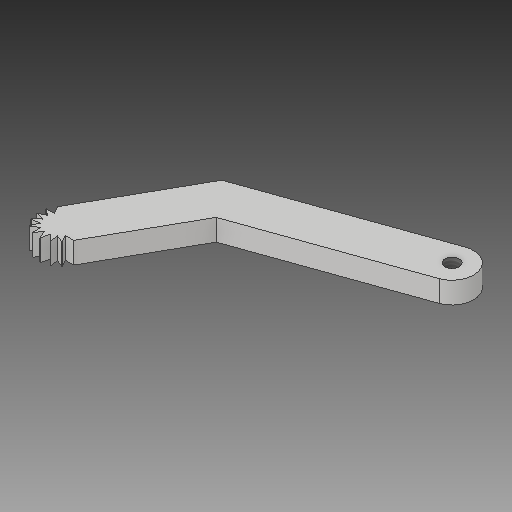
# Autodesk Inventor part: Finger
Saved by Autodesk Inventor 2017 (Build 210142000, 142)
## iProperties
Created: 2019-11-05
Part Number: Finger
Material: Generic
Document SubType Name: Modeling
Designer: asadb
Density: 1 g/cm^3
Appearance: Default
Mass: 3.76628 g
Surface Area: 24.9919 cm^2
Volume: 3.76628 cm^3
Author: asadb
Autodesk Inventor part; units mm, degrees
ref_plane "YZ Plane" through (0, 0, 0) normal (1, 0, 0) x (0, 1, 0)
ref_plane "XZ Plane" through (0, 0, 0) normal (0, 1, 0) x (-1, 0, 0)
ref_plane "XY Plane" through (0, 0, 0) normal (0, 0, 1) x (1, 0, 0)
sketch "Sketch1" plane through (0, 0, 0) normal (0, 1, 0) x (-1, 0, 0)
  line L0 (53.5, 38) -> (40.125, 14.25)
  line L1 (40.125, 14.25) -> (0, 0)
  line L2 (1.6733, -4.7117) -> (43.5628, 10.165)
  line L3 (43.5628, 10.165) -> (57.8567, 35.5465)
  line L4 (-1.6733, 4.7117) -> (36.6872, 18.335)
  line L5 (36.6872, 18.335) -> (49.1433, 40.4535)
  arc A0 (-1.6733, 4.7117) -> (1.6733, -4.7117) centre (0, 0) ccw
  arc A1 (57.8567, 35.5465) -> (49.1433, 40.4535) centre (53.5, 38) ccw
  dimension "d0" = 5
  dimension "d1" = 5
  dimension "d2" = 40.7078
  dimension "d3" = 5
  dimension "d4" = 25.3847
  dimension "d5" = 29.1297
  dimension "d6" = 53.5
  constraints: 12 end point, 4 point on circle, 3 coincident, 2 centre point, 1 tangent, 2 other
  measures "d0" distance between parallel lines of L1 L2
  measures "d1" distance between parallel lines of L1 L4
  measures "d2" distance of L4.start L4.end
  measures "d3" radius of A0
  measures "d4" distance of L4.end L5.end
  measures "d5" distance of L2.end L3.end
  measures "d6" horizontal distance of point (0, 0) A1.centre
extrude "Extrusion1" add sketch "Sketch1" along normal mid plane 5
sketch "Sketch2" plane through (0, 2.5, 0) normal (0, 1, 0) x (1, 0, 0)
  point P0 (0, 0)
  point P1 (0, 0)
  constraints: 1 coincident
hole "Hole1" at (0, 2.5, 0) direction (0, -1, 0) diameter 3.302 depth 12.3 tip angle 118 thread size "8-32 UNC" class "2B" standard "ANSI Unified Screw Threads"
sketch "Sketch3" plane through (0, 2.5, 0) normal (0, 1, 0) x (1, 0, 0)
  line L0 (-50.6525, -39.6036) -> (-48.6527, -39.5822)
  line L1 (-48.6527, -39.5822) -> (-49.634, -41.3248)
  line L2 (-49.634, -41.3248) -> (-50.6525, -39.6036)
  arc A0 (-57.8567, -35.5465) -> (-49.1433, -40.4535) centre (-53.5, -38) ccw projected
  line L3 (-49.1433, -40.4535) -> (-36.6872, -18.335) projected
  line L4 (-36.6872, -18.335) -> (-49.1433, -40.4535) projected
  line L5 (-49.1433, -40.4535) -> (-57.8567, -35.5465)
  line L6 (-51.4829, -40.5712) -> (-49.6271, -41.3167)
  line L7 (-49.6271, -41.3167) -> (-51.2007, -42.5512)
  line L8 (-51.2007, -42.5512) -> (-51.4829, -40.5712)
  line L9 (-52.6204, -41.1474) -> (-51.1912, -42.5463)
  line L10 (-51.1912, -42.5463) -> (-53.1174, -43.0846)
  line L11 (-53.1174, -43.0846) -> (-52.6204, -41.1474)
  line L12 (-53.8918, -41.2444) -> (-53.1067, -43.0838)
  line L13 (-53.1067, -43.0838) -> (-55.0923, -42.844)
  line L14 (-55.0923, -42.844) -> (-53.8918, -41.2444)
  line L15 (-55.1036, -40.8475) -> (-55.0822, -42.8473)
  line L16 (-55.0822, -42.8473) -> (-56.8248, -41.866)
  line L17 (-56.8248, -41.866) -> (-55.1036, -40.8475)
  line L18 (-56.0712, -40.0171) -> (-56.8167, -41.8729)
  line L19 (-56.8167, -41.8729) -> (-58.0512, -40.2993)
  line L20 (-58.0512, -40.2993) -> (-56.0712, -40.0171)
  line L21 (-56.6474, -38.8796) -> (-58.0463, -40.3088)
  line L22 (-58.0463, -40.3088) -> (-58.5846, -38.3826)
  line L23 (-58.5846, -38.3826) -> (-56.6474, -38.8796)
  line L24 (-56.7444, -37.6082) -> (-58.5838, -38.3933)
  line L25 (-58.5838, -38.3933) -> (-58.344, -36.4077)
  line L26 (-58.344, -36.4077) -> (-56.7444, -37.6082)
  line L27 (-56.3475, -36.3964) -> (-58.3473, -36.4178)
  line L28 (-58.3473, -36.4178) -> (-57.366, -34.6752)
  line L29 (-57.366, -34.6752) -> (-56.3475, -36.3964)
  point P0 (0, 0)
  point P1 (-49.6464, -40.1702)
  point P2 (-50.7702, -41.4797)
  point P3 (-52.3096, -42.2594)
  point P4 (-54.0303, -42.3907)
  point P5 (-55.6702, -41.8536)
  point P6 (-56.9797, -40.7298)
  point P7 (-57.7594, -39.1904)
  point P8 (-57.8907, -37.4697)
  point P9 (-57.3536, -35.8298)
  dimension "d16" = 2
  dimension "d19" = 180
  constraints: 56 end point, 2 perpendicular, 1 collinear, 1 point on line, 1 tangent, 64 other
  measures "d16" distance of L0.end L1.end
extrude "Extrusion2" cut sketch "Sketch3" against normal through all contours L5 A0 L2 | L0 L1 L5 | A0 L1 L2 | L27 A0 L5 | L5 L28 L29 | L7 A0 L6 | A0 L8 L6 | A0 L27 L28 | L7 L8 A0 | L26 A0 L25 | L26 L24 A0 | L10 A0 L9 | A0 L24 L25 | A0 L11 L9 | L10 L11 A0 | L23 A0 L22 | L13 A0 L12 | L23 L21 A0 | A0 L21 L22 | A0 L14 L12 | L13 L14 A0 | L20 A0 L19 | L16 A0 L15 | L20 L18 A0 | A0 L18 L19 | A0 L17 L15 | L16 L17 A0
body "Solid1"
